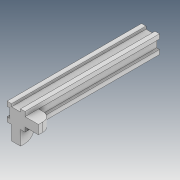
# Autodesk Inventor part: viga de suporte
Saved by Autodesk Inventor 2021 (Build 250183000, 183)
## iProperties
Created: 2020-09-22
Part Number: viga de suporte
Material: Genérico
Document SubType Name: Modeling
Designer: rapha
Density: 1 g/cm^3
Appearance: Padrão
Author: rapha
Autodesk Inventor part; units mm, degrees
ref_plane "YZ Plane" through (0, 0, 0) normal (1, 0, 0) x (0, 1, 0)
ref_plane "XZ Plane" through (0, 0, 0) normal (0, 1, 0) x (-1, 0, 0)
ref_plane "XY Plane" through (0, 0, 0) normal (0, 0, 1) x (1, 0, 0)
sketch "Esboço1" plane through (0, 0, 0) normal (0, 0, 1) x (1, 0, 0)
  line L0 (0, 0) -> (-5, 0)
  line L1 (-5, 0) -> (-5, -5)
  line L2 (-5, -5) -> (-2, -5)
  line L3 (-2, -5) -> (-2, -15)
  line L4 (-2, -15) -> (-5, -15)
  line L5 (-5, -15) -> (-5, -20)
  line L6 (-5, -20) -> (0, -20)
  line L7 (0, -20) -> (0, -17)
  line L8 (0, -17) -> (10, -17)
  line L9 (10, -17) -> (10, -20)
  line L10 (10, -20) -> (15, -20)
  line L11 (15, -20) -> (15, -15)
  line L12 (15, -15) -> (12, -15)
  line L13 (12, -15) -> (12, -5)
  line L14 (12, -5) -> (15, -5)
  line L15 (15, -5) -> (15, 0)
  line L16 (15, 0) -> (10, 0)
  line L17 (10, 0) -> (10, -3)
  line L18 (10, -3) -> (0, -3)
  line L19 (0, -3) -> (0, 0)
  dimension "d4" = 5
  dimension "d5" = 5
  dimension "d6" = 3
  dimension "d7" = 10
  dimension "d8" = 3
  dimension "d9" = 5
  dimension "d10" = 5
  dimension "d11" = 3
  dimension "d12" = 10
  dimension "d13" = 5
  dimension "d14" = 5
  dimension "d15" = 3
  dimension "d16" = 10
  dimension "d17" = 3
  dimension "d18" = 5
  dimension "d19" = 3
  dimension "d20" = 10
  constraints: 40 end point, 13 point on line, 8 perpendicular, 1 horizontal
  measures "d4" distance of L0.start L0.end
  measures "d5" distance of L0.end L1.end
  measures "d6" distance of L1.end L2.end
  measures "d7" distance of L2.end L3.end
  measures "d8" distance of L3.end L4.end
  measures "d9" distance of L4.end L5.end
  measures "d10" distance of L5.end L6.end
  measures "d11" distance of L6.end L7.end
  measures "d12" distance of L7.end L8.end
  measures "d13" distance of L9.end L10.end
  measures "d14" distance of L10.end L11.end
  measures "d15" distance of L11.end L12.end
  measures "d16" distance of L12.end L13.end
  measures "d17" distance of L13.end L14.end
  measures "d18" distance of L15.end L16.end
  measures "d19" distance of L16.end L17.end
  measures "d20" distance of L17.end L18.end
extrude "Extrusão1" add sketch "Esboço1" along normal blind 150
sketch "Esboço5" plane through (0, 0, 150) normal (0, 0, 1) x (1, 0, 0)
  line L0 (12, -15) -> (12, -5) projected
  line L1 (15, -15) -> (12, -15) projected
  line L2 (12, -5) -> (15, -5)
  line L3 (15, -5) -> (15, -15)
  line L4 (15, -15) -> (12, -15)
  line L5 (12, -15) -> (12, -5)
  line L6 (0, -17) -> (10, -17) projected
  line L7 (0, -17) -> (10, -17)
  line L8 (10, -17) -> (10, -20)
  line L9 (10, -20) -> (0, -20)
  line L10 (0, -20) -> (0, -17)
  line L11 (12, -5) -> (15, -5) projected
  line L12 (15, -5) -> (25, -5)
  line L13 (25, -5) -> (25, -15)
  line L14 (25, -15) -> (15, -15)
  line L15 (15, -15) -> (15, -5)
  line L16 (0, -20) -> (0, -17) projected
  line L17 (0, -20) -> (10, -20)
  line L18 (10, -20) -> (10, -31)
  line L19 (10, -31) -> (0, -31)
  line L20 (0, -31) -> (0, -20)
  line L21 (0, -31) -> (10, -31)
  line L22 (10, -31) -> (10, -36)
  line L23 (10, -36) -> (0, -36)
  line L24 (0, -36) -> (0, -31)
  line L25 (25, -5) -> (30, -5)
  line L26 (30, -5) -> (30, -15)
  line L27 (30, -15) -> (25, -15)
  line L28 (25, -15) -> (25, -5)
  point P0 (0, 0)
  constraints: 48 end point, 12 parallel, 6 horizontal, 6 perpendicular, 1 point on line
extrude "Extrusão2" add sketch "Esboço5" against normal blind 15
fillet "Arredondamento1" radius 10 2 edges at (30, -10, 135) (5, -36, 135)
